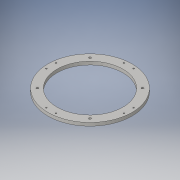
# Autodesk Inventor part: fixedRing
Saved by Autodesk Inventor 2016 SP1 (Build 200210100, 210)
## iProperties
Created: 2016-01-13
Part Number: fixedRing
Material: Generic
Document SubType Name: Modeling
Designer: ddeboer
Density: 1 g/cm^3
Appearance: Default
Author: ddeboer
Autodesk Inventor part; units mm, degrees
ref_plane "YZ Plane" through (0, 0, 0) normal (1, 0, 0) x (0, 1, 0)
ref_plane "XZ Plane" through (0, 0, 0) normal (0, 1, 0) x (-1, 0, 0)
ref_plane "XY Plane" through (0, 0, 0) normal (0, 0, 1) x (1, 0, 0)
sketch "Sketch1" plane through (0, 0, 0) normal (0, 1, 0) x (-1, 0, 0)
  circle A0 centre (0, 0) radius 165.1
  circle A1 centre (0, 0) radius 129.54
  dimension "d0" = 330.2
  dimension "d1" = 259.08
  constraints: 2 centre point, 2 coincident
  measures "d0" diameter of A0
  measures "d1" diameter of A1
extrude "Extrusion1" add sketch "Sketch1" along normal blind 12.7
sketch "Sketch2" plane through (0, 12.7, 0) normal (0, 1, 0) x (1, 0, 0)
  circle A0 centre (19.05, -152.4) radius 4.7802
  line L0 (0, 0) -> (0, -55.3703) construction
  circle A1 centre (-19.05, -152.4) radius 4.7802
  dimension "d6" = 152.4
  dimension "d7" = 19.05
  constraints: 2 centre point, 2 end point, 1 symmetric about line, 1 vertical, 1 other
  measures "d6" vertical distance of L0.start A0.centre
  measures "d7" horizontal distance of L0.start A0.centre
hole "Hole1" at (19.05, 12.7, 152.4) at (-19.05, 12.7, 152.4) direction (0, -1, 0) diameter 5.3594 depth 17.2466 tip angle 118 thread size "1/4-28 UNF" class "2B" standard "ANSI Unified Screw Threads"
pattern_circular "Circular Pattern1" count 4 over 360 about axis through (0, -10, 0) along (0, 1, 0) of "Hole1"
sketch "Sketch3" plane through (0, 12.7, 0) normal (0, 1, 0) x (1, 0, 0)
  line L0 (0, 0) -> (103.2729, 103.2729) construction
  line L1 (0, 0) -> (146.05, 0) construction
  circle A0 centre (103.2729, 103.2729) radius 4.2786
  dimension "d18" = 146.05
  dimension "d19" = 45
  constraints: 4 end point, 1 centre point, 1 coincident, 1 equal length, 1 horizontal
  measures "d18" distance of L0.start L0.end
  measures "d19" angle of L1 L0
hole "Hole2" at (103.2729, 12.7, -103.2729) direction (0, -1, 0) diameter 8.4328 end through all clearance for "Flat Head Machine Screw (82)" size "5/16" standard "Ansi Unified Screw Threads"
pattern_circular "Circular Pattern2" count 4 over 360 about axis through (0, 0, 0) along (0, 1, 0) of "Hole2"
body "Solid1"
